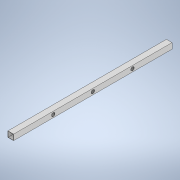
# Autodesk Inventor part: 1x1 28in WChurro Holes
Saved by Autodesk Inventor 2020 (Build 240168000, 168)
## iProperties
Created: 2020-01-14
Part Number: 1x1 28in WChurro Holes
Material: Generic
Document SubType Name: Modeling
Designer: aidan
Density: 1 g/cm^3
Appearance: Default
Author: aidan
Autodesk Inventor part; units mm, degrees
ref_plane "YZ Plane" through (0, 0, 0) normal (1, 0, 0) x (0, 1, 0)
ref_plane "XZ Plane" through (0, 0, 0) normal (0, 1, 0) x (-1, 0, 0)
ref_plane "XY Plane" through (0, 0, 0) normal (0, 0, 1) x (1, 0, 0)
sketch "Sketch1" plane through (0, 0, 0) normal (0, 0, 1) x (1, 0, 0)
  line L0 (-14.0074, 10.2243) -> (11.3926, 10.2243)
  line L1 (11.3926, 10.2243) -> (11.3926, -15.1757)
  line L2 (11.3926, -15.1757) -> (-14.0074, -15.1757)
  line L3 (-14.0074, -15.1757) -> (-14.0074, 10.2243)
  line L4 (10.1226, 8.9543) -> (-12.7374, 8.9543)
  line L5 (-12.7374, 8.9543) -> (-12.7374, -13.9057)
  line L6 (-12.7374, -13.9057) -> (10.1226, -13.9057)
  line L7 (10.1226, -13.9057) -> (10.1226, 8.9543)
  point P0 (0, 0)
  dimension "d0" = 25.4
  dimension "d1" = 1.27
  constraints: 16 end point, 4 parallel, 3 perpendicular, 1 horizontal, 3 other
  measures "d0" distance of L0.start L0.end
  measures "d1" distance between parallel lines of L0 L4
extrude "Extrusion1" add sketch "Sketch1" along normal blind 711.2
sketch "Sketch2" plane through (11.3926, -15.1757, 0) normal (1, 0, 0) x (0, 0, -1)
  circle A0 centre (-355.6, 12.7) radius 7.9375
  line L0 (-711.2, 1.27) -> (-711.2, 24.13) projected
  line L1 (-711.2, 12.7) -> (0, 12.7) construction
  line L2 (0, 25.4) -> (0, 0) projected
  circle A1 centre (-533.4, 12.7) radius 7.9375
  circle A2 centre (-177.8, 12.7) radius 7.9375
  point P0 (0, 15.1757)
  dimension "d5" = 15.875
  dimension "d6" = 177.8
  dimension "d7" = 177.8
  dimension "d8" = 355.6
  constraints: 3 centre point, 3 midpoint, 2 end point, 2 equal radius, 2 point on line
  measures "d5" diameter of A0
  measures "d6" distance from line of L0 A1.centre
  measures "d7" distance from line of L2 A2.centre
  measures "d8" horizontal distance of L0.end A0.centre
extrude "Extrusion2" cut sketch "Sketch2" against normal blind 2.54
sketch "Sketch3" plane through (-14.0074, -15.1757, 0) normal (-1, 0, 0) x (0, 0, 1)
  circle A0 centre (177.8, 12.7) radius 7.9375 construction
  circle A1 centre (355.6, 12.7) radius 7.9375 construction
  circle A2 centre (533.4, 12.7) radius 7.9375 construction
  circle A3 centre (177.8, 12.7) radius 2.9972
  circle A4 centre (355.6, 12.7) radius 2.9972
  circle A5 centre (533.4, 12.7) radius 2.9972
  point P0 (0, 15.1757)
  dimension "d11" = 5.9944
  constraints: 3 centre point, 3 coincident, 2 equal radius
  measures "d11" diameter of A3
extrude "Extrusion3" cut sketch "Sketch3" against normal blind 2.54
equation "\"d6\" = d4"
equation "\"d7\" = d4"
equation "\"d8\" = 0.5 * d2"
equation "\"d4\" = 177.8"
equation "\"d2\" = 711.2"
body "Solid1"
